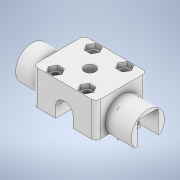
# Autodesk Inventor part: Part8
Saved by Autodesk Inventor 2022 (Build 260153000, 153)
## iProperties
Created: 2022-12-25
Part Number: Part8
Material: ABS Plastic
Document SubType Name: Modeling
Designer: Kamil
Density: 1.06 g/cm^3
Appearance: Smooth - White
Author: Kamil
Autodesk Inventor part; units mm, degrees
ref_plane "YZ Plane" through (0, 0, 0) normal (1, 0, 0) x (0, 1, 0)
ref_plane "XZ Plane" through (0, 0, 0) normal (0, 1, 0) x (-1, 0, 0)
ref_plane "XY Plane" through (0, 0, 0) normal (0, 0, 1) x (1, 0, 0)
ref_plane "Work Plane1" through (88.6183, 20.8479, 68.1697) normal (-1, 0, 0) x (0, 1, 0)
sketch "Sketch1" plane through (88.6183, 20.8479, 68.1697) normal (-1, 0, 0) x (0, 1, 0)
  arc A0 (4.3225, -4.9221) -> (4.3225, 4.9221) centre (-2.06, 0) ccw
  arc A1 (4.3225, -4.9221) -> (4.3225, 4.9221) centre (-2.06, 0) ccw
  arc A2 (4.3225, -4.9221) -> (4.3225, 4.9221) centre (-2.06, 0) ccw
  line L0 (-4.065, 4.6) -> (4.065, 4.6)
  arc A3 (4.065, -4.6) -> (4.065, 4.6) centre (-2.06, 0) ccw
  line L1 (4.065, -4.6) -> (-4.065, -4.6)
  arc A4 (-4.065, 4.6) -> (-4.065, -4.6) centre (2.06, 0) ccw
  circle A5 centre (0, 0) radius 1
  arc A6 (4.3225, -4.9221) -> (4.3225, 4.9221) centre (-2.06, 0) ccw
  arc A7 (4.3225, -4.9221) -> (4.3225, 4.9221) centre (-2.06, 0) ccw
  line L2 (-4.1641, 5) -> (4.1641, 5)
  arc A8 (5.9696, 0.6989) -> (4.3225, 4.9221) centre (-2.06, 0) ccw
  arc A9 (4.3225, 4.9221) -> (4.1641, 5) centre (4.1641, 4.8) ccw
  spline S0 degree 3 poles (-4.1641, 5) (-4.1596, 4.9818) (-4.1529, 4.9545) (-4.1346, 4.8801) (-4.1163, 4.8058) (-4.0908, 4.7033) (-4.065, 4.6) knots 0 0 0 0 0.5 0.5 0.5 1 1 1 1
  arc A10 (-4.3225, 4.9221) -> (-5.9696, 0.6989) centre (2.06, 0) ccw
  arc A11 (-4.1641, 5) -> (-4.3225, 4.9221) centre (-4.1641, 4.8) ccw
  line L3 (4.1641, -5) -> (-4.1641, -5)
  arc A12 (4.1641, -5) -> (4.3225, -4.9221) centre (4.1641, -4.8) ccw
  arc A13 (4.3225, -4.9221) -> (5.9244, -1.1011) centre (-2.06, 0) ccw
  arc A14 (-5.9244, -1.1011) -> (-4.3225, -4.9221) centre (2.06, 0) ccw
  arc A15 (-4.3225, -4.9221) -> (-4.1641, -5) centre (-4.1641, -4.8) ccw
  arc A16 (-5.9696, 0.6989) -> (-5.9244, -1.1011) centre (2.06, 0) ccw
  circle A17 centre (0, 0) radius 9.5
  line L4 (9.5, 0) -> (8.5, 0)
  line L5 (-6, 4) -> (-6, -4)
  arc A18 (-6, -4) -> (-5, -5) centre (-5, -4) ccw
  line L6 (-5, -5) -> (5, -5)
  arc A19 (5, -5) -> (6, -4) centre (5, -4) ccw
  line L7 (6, -4) -> (6, 4)
  arc A20 (6, 4) -> (5, 5) centre (5, 4) ccw
  line L8 (5, 5) -> (-5, 5)
  arc A21 (-5, 5) -> (-6, 4) centre (-5, 4) ccw
  circle A22 centre (-3, -2.5) radius 0.5
  circle A23 centre (0, 0) radius 0.5329
  line L9 (6, 4) -> (6, -4)
  arc A24 (6, 4) -> (5, 5) centre (5, 4) ccw
  line L10 (-5, 5) -> (5, 5)
  arc A25 (-5, 5) -> (-6, 4) centre (-5, 4) ccw
  line L11 (-6, -4) -> (-6, 4)
  arc A26 (-6, -4) -> (-5, -5) centre (-5, -4) ccw
  line L12 (5, -5) -> (-5, -5)
  arc A27 (5, -5) -> (6, -4) centre (5, -4) ccw
  circle A28 centre (0, 0) radius 1.5
  circle A29 centre (3.5, -2.5) radius 1.5
  circle A30 centre (-3.5, 2.5) radius 1.5
  circle A31 centre (4.5, 0) radius 0.625
  circle A32 centre (-4.5, 0) radius 0.625
  circle A33 centre (0, 0) radius 8.5
  line L13 (6, 4) -> (7.5, 4)
  line L14 (6, -4) -> (7.5, -4)
  line L15 (0, -9.5) -> (0, -7.9)
  circle A34 centre (0, 0) radius 7.9
  line L16 (5, -5) -> (5, -6.1164)
  line L17 (-5, -5) -> (-5, -6.1164)
  line L18 (-5, 5) -> (-5, 6.1164)
  line L19 (5, 5) -> (5, 6.1164)
  point P0 (-20.8479, 68.1697)
  point P1 (6.8125, -4)
  point P2 (6.8125, 4)
  dimension "d0" = 1
  dimension "d1" = 1.6
  constraints: 16 end point, 10 point on circle, 2 centre point, 2 coincident, 2 horizontal, 2 point on line, 2 vertical, 1 parallel
  measures "d0" distance of L4.start L4.end
  measures "d1" distance of L15.start L15.end
extrude "Extrusion1" add sketch "Sketch1" along normal blind 5 contours L6 L16 A34 L17 L3 | L7 L13 A34 L14 | L8 L2 L18 A34 L19
sketch "Sketch2" plane through (88.6183, 20.8479, 68.1697) normal (1, 0, 0) x (0, 0, -1)
  arc A0 (-6.1164, 5) -> (-6.1164, -5) centre (0, 0) ccw projected
  line L0 (-5, -5) -> (-6.1164, -5) projected
  line L1 (-5, 5) -> (-5, -5) projected
  line L2 (-6.1164, 5) -> (-5, 5) projected
  line L3 (4, 6.8125) -> (4, 6) projected
  arc A1 (4, 6.8125) -> (-4, 6.8125) centre (0, 0) ccw projected
  line L4 (-4, 6) -> (-4, 6.8125) projected
  line L5 (4, 6) -> (-4, 6) projected
  arc A2 (6.1164, -5) -> (6.1164, 5) centre (0, 0) ccw projected
  line L6 (5, 5) -> (6.1164, 5) projected
  line L7 (5, -5) -> (5, 5) projected
  line L8 (6.1164, -5) -> (5, -5) projected
  circle A3 centre (0, 0) radius 7.9
  line L9 (5, -5) -> (5, 5) projected
  arc A4 (5, 5) -> (4, 6) centre (4, 5) ccw projected
  line L10 (4, 6) -> (-4, 6) projected
  arc A5 (-4, 6) -> (-5, 5) centre (-4, 5) ccw projected
  line L11 (-5, 5) -> (-5, -5) projected
  arc A6 (-5, -5) -> (-4, -6) centre (-4, -5) ccw projected
  line L12 (-4, -6) -> (4, -6) projected
  arc A7 (4, -6) -> (5, -5) centre (4, -5) ccw projected
  circle A8 centre (2.5, -3.5) radius 1.75 projected
  circle A9 centre (-2.5, 3.5) radius 1.75 projected
  circle A10 centre (0, -4.5) radius 0.625 projected
  circle A11 centre (0, 4.5) radius 0.625 projected
  circle A12 centre (0, 0) radius 2 projected
  point P0 (68.1697, -20.8479)
  point P1 (6.1164, 5)
  point P2 (-4, 6.8125)
  constraints: 1 centre point, 1 coincident
ref_plane "Work Plane2" through (97.6183, 14.8479, 63.1697) normal (1, 0, 0) x (0, 1, 0)
extrude "Extrusion2" add sketch "Sketch2" along normal up to surface (9 mm away) contours L2 L1 L0 A0 | A3 L4 A5 L2 | A1 L3 L5 L4 | L8 L7 L6 A2 | A3 L6 A4 L3
sketch "Sketch3" plane through (83.6183, 20.8479, 68.1697) normal (-1, 0, 0) x (0, 0, 1)
  line L0 (6.1164, 5) -> (5, 5) projected
  arc A0 (6.1164, 5) -> (4, 6.8125) centre (0, 0) ccw projected
  line L1 (4, 6) -> (4, 6.8125) projected
  arc A1 (5, 5) -> (4, 6) centre (4, 5) ccw projected
  line L2 (-4, 6.8125) -> (-4, 6) projected
  arc A2 (-4, 6.8125) -> (-6.1164, 5) centre (0, 0) ccw projected
  line L3 (-5, 5) -> (-6.1164, 5) projected
  arc A3 (-4, 6) -> (-5, 5) centre (-4, 5) ccw projected
  point P0 (-68.1697, -20.8479)
extrude "Extrusion3" add sketch "Sketch3" against normal blind 10
sketch "Sketch4" plane through (88.6183, 20.8479, 68.1697) normal (-1, 0, 0) x (0, 1, 0)
  arc A0 (5.9696, 0.6989) -> (4.3225, 4.9221) centre (-2.06, 0) ccw projected
  arc A1 (4.3225, -4.9221) -> (5.9244, -1.1011) centre (-2.06, 0) ccw projected
  line L0 (4.1641, -5) -> (-4.1641, -5) projected
  line L1 (4.5, -1.1011) -> (4.5, 0.6989) projected
  line L2 (4.5, 0.6989) -> (5.9696, 0.6989) projected
  arc A2 (5.9696, 0.6989) -> (4.3225, 4.9221) centre (-2.06, 0) ccw projected
  arc A3 (4.3225, 4.9221) -> (4.1641, 5) centre (4.1641, 4.8) ccw projected
  line L3 (1, 5) -> (4.1641, 5) projected
  line L4 (1, 5) -> (1, -5) projected
  line L5 (1, -5) -> (4.1641, -5) projected
  arc A4 (4.1641, -5) -> (4.3225, -4.9221) centre (4.1641, -4.8) ccw projected
  arc A5 (4.3225, -4.9221) -> (5.9244, -1.1011) centre (-2.06, 0) ccw projected
  line L6 (5.9244, -1.1011) -> (4.5, -1.1011) projected
  arc A6 (-5, -6.1164) -> (-5, 6.1164) centre (0, 0) ccw projected
  line L7 (-5, 6.1164) -> (-5, 5) projected
  line L8 (-5, 5) -> (5, 5) projected
  arc A7 (6, 4) -> (5, 5) centre (5, 4) ccw projected
  line L9 (6, 4) -> (6, -4) projected
  arc A8 (5, -5) -> (6, -4) centre (5, -4) ccw projected
  line L10 (5, -5) -> (-5, -5) projected
  line L11 (-5, -5) -> (-5, -6.1164) projected
  arc A9 (5.9244, -1.1011) -> (5.9696, 0.6989) centre (-2.06, 0) ccw projected
  arc A10 (-4.3225, 4.9221) -> (-5.9696, 0.6989) centre (2.06, 0) ccw projected
  arc A11 (-5.9244, -1.1011) -> (-4.3225, -4.9221) centre (2.06, 0) ccw projected
  arc A12 (-5.9696, 0.6989) -> (-5.9244, -1.1011) centre (2.06, 0) ccw projected
  line L12 (-4.5, 0.6989) -> (-4.5, -1.1011) projected
  line L13 (-4.5, -1.1011) -> (-5.9244, -1.1011) projected
  arc A13 (-5.9244, -1.1011) -> (-4.3225, -4.9221) centre (2.06, 0) ccw projected
  arc A14 (-4.3225, -4.9221) -> (-4.1641, -5) centre (-4.1641, -4.8) ccw projected
  line L14 (-4.1641, -5) -> (-1, -5) projected
  line L15 (-1, 5) -> (-1, -5) projected
  line L16 (-4.1641, 5) -> (-1, 5) projected
  arc A15 (-4.1641, 5) -> (-4.3225, 4.9221) centre (-4.1641, 4.8) ccw projected
  arc A16 (-4.3225, 4.9221) -> (-5.9696, 0.6989) centre (2.06, 0) ccw projected
  line L17 (-5.9696, 0.6989) -> (-4.5, 0.6989) projected
  line L18 (-5, 5) -> (-5, -6.1164)
  point P0 (-20.8479, 68.1697)
  point P1 (-5, 3.8885)
  point P2 (-5, -3.8885)
  point P3 (-5, -5)
  point P4 (-4.1641, -5)
  point P5 (6, 0)
  point P6 (4.1641, 5)
  constraints: 2 end point
extrude "Extrusion4" add sketch "Sketch4" along normal up to surface (5 mm away) contours A0 A3 L8 A7 L9 A9 | L9 A8 L10 A4 A1 A9 | A15 A10 L18 L8 | L10 L18 A11 A14
ref_plane "Work Plane3" through (70.1183, 20.8479, 68.3708) normal (-1, 0, 0) x (0, 1, 0)
sketch "Sketch5" plane through (97.6183, 26.8479, 64.1697) normal (0, -1, 0) x (1, 0, 0)
  line L0 (-5.5, 8) -> (-5.5, 0) projected
  line L1 (-5.5, 8) -> (-4.5, 8) projected
  line L2 (-4.5, 8) -> (-4.5, 0) projected
  line L3 (-4.5, 0) -> (-5.5, 0) projected
  line L4 (-8, 0) -> (-8, 8) projected
  line L5 (-8, 8) -> (-9, 8) projected
  line L6 (-9, 0) -> (-9, 8) projected
  line L7 (-9, 0) -> (-8, 0) projected
  line L8 (-1, 8) -> (-1, 0) projected
  line L9 (-1, 0) -> (0, 0) projected
  line L10 (0, 8) -> (0, 0) projected
  line L11 (0, 8) -> (-1, 8) projected
  line L12 (0, 0) -> (-9, 0) projected
  line L13 (-5.6036, 0) -> (-7.8841, 0)
  line L14 (-7.8841, 0) -> (-7.8841, 1)
  line L15 (-7.8841, 1) -> (-5.6036, 1)
  line L16 (-5.6036, 1) -> (-5.6036, 0)
  line L17 (0, 8) -> (-9, 8) projected
  line L18 (-5.6036, 8) -> (-7.8841, 8)
  line L19 (-7.8841, 8) -> (-7.8841, 7)
  line L20 (-7.8841, 7) -> (-5.6036, 7)
  line L21 (-5.6036, 7) -> (-5.6036, 8)
  line L22 (-1.16, 0) -> (-4.2946, 0)
  line L23 (-4.2946, 0) -> (-4.2946, 1)
  line L24 (-4.2946, 1) -> (-1.16, 1)
  line L25 (-1.16, 1) -> (-1.16, 0)
  line L26 (-1.16, 8) -> (-4.2946, 8)
  line L27 (-4.2946, 8) -> (-4.2946, 7)
  line L28 (-4.2946, 7) -> (-1.16, 7)
  line L29 (-1.16, 7) -> (-1.16, 8)
  line L30 (0, -2.1164) -> (-14, -2.1164) projected
  line L31 (-1.16, 1) -> (-4.2946, 1)
  line L32 (-4.2946, 1) -> (-4.2946, -2.1164)
  line L33 (-4.2946, -2.1164) -> (-1.16, -2.1164)
  line L34 (-1.16, -2.1164) -> (-1.16, 1)
  line L35 (-5.6036, 1) -> (-7.8841, 1)
  line L36 (-7.8841, 1) -> (-7.8841, -2.1164)
  line L37 (-7.8841, -2.1164) -> (-5.6036, -2.1164)
  line L38 (-5.6036, -2.1164) -> (-5.6036, 1)
  line L39 (-14, 10.1164) -> (0, 10.1164) projected
  line L40 (-5.6036, 7) -> (-7.8841, 7)
  line L41 (-7.8841, 7) -> (-7.8841, 10.1164)
  line L42 (-7.8841, 10.1164) -> (-5.6036, 10.1164)
  line L43 (-5.6036, 10.1164) -> (-5.6036, 7)
  line L44 (-1.16, 7) -> (-4.2946, 7)
  line L45 (-4.2946, 7) -> (-4.2946, 10.1164)
  line L46 (-4.2946, 10.1164) -> (-1.16, 10.1164)
  line L47 (-1.16, 10.1164) -> (-1.16, 7)
  point P0 (-97.6183, -64.1697)
  point P1 (-1.16, 8)
  point P2 (-1.16, 10.1164)
  point P3 (-4.2946, 8)
  point P4 (-5.6036, 0)
  point P5 (-7.8841, 0)
  point P6 (-1.16, -2.1164)
  point P7 (-1.16, 0)
  point P8 (-4.2946, 0)
  dimension "d10" = 1
  dimension "d11" = 1
  constraints: 64 end point, 16 parallel, 10 point on line, 8 horizontal, 8 perpendicular
  measures "d10" distance between parallel lines of L12 L15
  measures "d11" distance of L19.end L18.end
extrude "Extrusion5" add sketch "Sketch5" along normal blind 0.5 contours L21 L20 L19 L17 | L17 L41 L39 L43 | L38 L30 L36 L12 | L12 L14 L15 L16 | L45 L39 L47 L17 | L17 L29 L28 L27 | L23 L24 L25 L12 | L12 L34 L30 L32
sketch "Sketch6" plane through (97.6183, 15.8479, 63.1697) normal (1, 0, 0) x (0, 0, -1)
  arc A0 (-9, 11) -> (-10, 10) centre (-9, 10) ccw projected
  line L0 (-1, 11) -> (-9, 11) projected
  arc A1 (0, 10) -> (-1, 11) centre (-1, 10) ccw projected
  line L1 (0, 0) -> (0, 10) projected
  line L2 (1.1164, 0) -> (0, 0) projected
  arc A2 (1.1164, 0) -> (-11.1164, 0) centre (-5, 5) ccw projected
  line L3 (-10, 0) -> (-11.1164, 0) projected
  line L4 (-10, 10) -> (-10, 0) projected
  arc A3 (-10.1391, 11) -> (-10.671, 10.5) centre (-5, 5) ccw projected
  line L5 (-10.1391, 11) -> (-11.1164, 11) projected
  line L6 (-11.1164, 11) -> (-11.1164, 10.5) projected
  line L7 (-10.671, 10.5) -> (-11.1164, 10.5) projected
  arc A4 (0.671, 10.5) -> (0.1391, 11) centre (-5, 5) ccw projected
  line L8 (1.1164, 10.5) -> (0.671, 10.5) projected
  line L9 (1.1164, 11) -> (1.1164, 10.5) projected
  line L10 (1.1164, 11) -> (0.1391, 11) projected
  point P0 (63.1697, -15.8479)
  point P1 (0.1391, 11)
  point P2 (0.671, 10.5)
  point P3 (-10.671, 10.5)
  point P4 (-10.1391, 11)
extrude "Extrusion6" cut sketch "Sketch6" against normal through all contours L7 L6 L5 A2 | A2 L10 L9 L8
sketch "Sketch7" plane through (83.6183, 20.8479, 68.1697) normal (-1, 0, 0) x (0, 0, 1)
  arc A0 (6.1164, -5) -> (-6.1164, -5) centre (0, 0) ccw projected
  line L0 (-6.1164, -5) -> (-3.8885, -5) projected
  arc A1 (-4.9221, -4.3225) -> (-3.8885, -5) centre (0, 2.06) ccw projected
  arc A2 (-5, -4.1641) -> (-4.9221, -4.3225) centre (-4.8, -4.1641) ccw projected
  line L1 (-5, -4.1641) -> (-5, 4.1641) projected
  arc A3 (-4.9221, 4.3225) -> (-5, 4.1641) centre (-4.8, 4.1641) ccw projected
  arc A4 (4.9221, 4.3225) -> (-4.9221, 4.3225) centre (0, -2.06) ccw projected
  arc A5 (5, 4.1641) -> (4.9221, 4.3225) centre (4.8, 4.1641) ccw projected
  line L2 (5, 4.1641) -> (5, -4.1641) projected
  arc A6 (4.9221, -4.3225) -> (5, -4.1641) centre (4.8, -4.1641) ccw projected
  arc A7 (3.8885, -5) -> (4.9221, -4.3225) centre (0, 2.06) ccw projected
  line L3 (6.1164, -5) -> (3.8885, -5) projected
  point P0 (-68.1697, -20.8479)
extrude "Extrusion7" cut sketch "Sketch7" against normal blind 1.5
sketch "Sketch8" plane through (85.1183, 20.8479, 68.1697) normal (-1, 0, 0) x (0, 0, 1)
  arc A0 (6.1164, -5) -> (-6.1164, -5) centre (0, 0) ccw projected
  line L0 (-3.8885, -5) -> (-6.1164, -5) projected
  arc A1 (-4.9221, -4.3225) -> (-3.8885, -5) centre (0, 2.06) ccw projected
  arc A2 (-5, -4.1641) -> (-4.9221, -4.3225) centre (-4.8, -4.1641) ccw projected
  line L1 (-5, 4.1641) -> (-5, -4.1641) projected
  arc A3 (-4.9221, 4.3225) -> (-5, 4.1641) centre (-4.8, 4.1641) ccw projected
  arc A4 (4.9221, 4.3225) -> (-4.9221, 4.3225) centre (0, -2.06) ccw projected
  arc A5 (5, 4.1641) -> (4.9221, 4.3225) centre (4.8, 4.1641) ccw projected
  line L2 (5, -4.1641) -> (5, 4.1641) projected
  arc A6 (4.9221, -4.3225) -> (5, -4.1641) centre (4.8, -4.1641) ccw projected
  arc A7 (3.8885, -5) -> (4.9221, -4.3225) centre (0, 2.06) ccw projected
  line L3 (6.1164, -5) -> (3.8885, -5) projected
  circle A8 centre (0, 0) radius 12.5 projected
  circle A9 centre (0, 0) radius 9.5 projected
  circle A10 centre (0, 0) radius 16.1 projected
  line L4 (-5, 4.1641) -> (-5, -4.1641) projected
  line L5 (-5, 0) -> (-8, 0)
  line L6 (-8, 0) -> (-8, 11.4896)
  line L7 (5, 0) -> (8, 0)
  arc A11 (4.9221, 4.3225) -> (0, 6) centre (0, -2.06) ccw projected
  line L8 (0, 6) -> (0, 9)
  line L9 (0, 9) -> (-8, 9)
  line L10 (8, 0) -> (8, 9.5)
  line L11 (0, 9) -> (8, 9)
  line L12 (-6.1164, -5) -> (6.1164, -5)
  line L13 (-6.1164, -5) -> (-10.7059, -5)
  line L14 (-10.7059, -5) -> (9.6672, -5)
  line L15 (-8, -1.0781) -> (-8, -5.1235)
  line L16 (8, 0) -> (8.0777, -5)
  line L17 (-8, 0) -> (-8, -1.0781)
  point P0 (-68.1697, -20.8479)
  point P1 (-8, -5)
  dimension "d18" = 3
  dimension "d19" = 3
  dimension "d20" = 3
  constraints: 26 end point, 6 point on line, 4 perpendicular, 3 horizontal, 2 midpoint, 2 point on circle, 2 vertical
  measures "d18" distance of L5.start L5.end
  measures "d19" distance of L7.start L7.end
  measures "d20" distance of L8.start L8.end
extrude "Extrusion8" add sketch "Sketch8" along normal up to surface (15 mm away) contours L3 A7 A6 L2 L7 A0 | A0 L7 L16 L14 | L7 L2 A5 A4 L8 A0 | A0 L8 L11 A9 L10 L7 | L8 A4 A3 L1 L5 A0 | A0 L5 L6 A9 L9 L8 | L0 A0 L5 L1 A2 A1 | A0 L13 L15 L17 L5 | A9 L11 L10 | A9 L6 L9
sketch "Sketch9" plane through (85.1183, 15.8479, 60.1697) normal (0, 0, -1) x (-1, 0, 0)
  line L0 (15, 0) -> (15, 14) projected
  line L1 (0, 14) -> (15, 14) projected
  line L2 (0, 14) -> (0, 0) projected
  line L3 (0, 0) -> (15, 0) projected
  point P0 (85.1183, -15.8479)
extrude "Extrusion9" add sketch "Sketch9" along normal blind 5
sketch "Sketch10" plane through (85.1183, 20.8479, 76.1697) normal (0, 0, 1) x (1, 0, 0)
  line L0 (-15, 9) -> (-15, 0) projected
  line L1 (0, 0) -> (-15, 0) projected
  line L2 (0, 0) -> (0, 9) projected
  line L3 (0, 9) -> (-15, 9) projected
  line L4 (-15, 0) -> (-15, -5) projected
  line L5 (0, -5) -> (-15, -5) projected
  line L6 (0, -5) -> (0, 0) projected
  line L7 (0, 0) -> (-15, 0) projected
  point P0 (-85.1183, -20.8479)
  point P1 (-15, 0)
extrude "Extrusion10" add sketch "Sketch10" along normal blind 5
sketch "Sketch11" plane through (70.1183, 29.8479, 55.1697) normal (0, 1, 0) x (1, 0, 0)
  line L0 (0, -8) -> (18.5, -8) projected
  line L1 (27.5, -8) -> (18.5, -8) projected
  line L2 (27.5, -8) -> (18.5, -8) projected
  line L3 (0, -8) -> (18.5, -8) projected
  line L4 (0, -18) -> (18.5, -18) projected
  line L5 (27.5, -18) -> (18.5, -18) projected
  line L6 (27.5, -18) -> (18.5, -18) projected
  line L7 (0, -18) -> (18.5, -18) projected
  line L8 (0, 0) -> (0, -26) projected
  line L9 (15, -26) -> (0, -26) projected
  line L10 (15, 0) -> (15, -26) projected
  line L11 (0, 0) -> (15, 0) projected
  line L12 (15, 0) -> (0, 0) projected
  line L13 (7.5, 0) -> (7.5, -8)
  line L14 (18.5, -17.9221) -> (0, -17.9221) projected
  circle A0 centre (7.5, -4) radius 1.65
  line L15 (15, 0) -> (15, -26) projected
  line L16 (0, -9.1115) -> (0, 0) projected
  line L17 (15, 0) -> (0, 0)
  line L18 (0, 0) -> (0, -0.3)
  line L19 (0, -0.3) -> (15, -0.3)
  line L20 (15, -0.3) -> (15, 0)
  line L21 (7.5, -4) -> (7.5, -0.8)
  line L22 (7.5, -0.8) -> (7.5, -7.2)
  line L23 (5.6525, -7.2) -> (3.805, -4)
  line L24 (3.805, -4) -> (5.6525, -0.8)
  line L25 (5.6525, -0.8) -> (9.3475, -0.8)
  line L26 (9.3475, -0.8) -> (11.195, -4)
  line L27 (11.195, -4) -> (9.3475, -7.2)
  line L28 (9.3475, -7.2) -> (5.6525, -7.2)
  line L29 (15, 0) -> (0, 0)
  line L30 (0, 0) -> (0, -0.8)
  line L31 (0, -0.8) -> (15, -0.8)
  line L32 (15, -0.8) -> (15, 0)
  line L33 (0, -26) -> (15, -26) projected
  line L34 (7.5, -26) -> (7.5, -18)
  line L35 (0, -18) -> (18.5, -18) projected
  circle A1 centre (7.5, -22) radius 1.65
  line L36 (3.805, -22) -> (5.6525, -18.8)
  line L37 (5.6525, -18.8) -> (9.3475, -18.8)
  line L38 (9.3475, -18.8) -> (11.195, -22)
  line L39 (11.195, -22) -> (9.3475, -25.2)
  line L40 (9.3475, -25.2) -> (5.6525, -25.2)
  line L41 (5.6525, -25.2) -> (3.805, -22)
  line L42 (0, -16.8885) -> (0, -26) projected
  line L43 (0, -26) -> (15, -26)
  line L44 (15, -26) -> (15, -25.2)
  line L45 (15, -25.2) -> (0, -25.2)
  line L46 (0, -25.2) -> (0, -26)
  point P0 (-70.1183, 55.1697)
  point P1 (9.3475, -0.8)
  point P2 (15, -0.8)
  point P3 (0, -0.8)
  point P4 (5.6525, -0.8)
  point P5 (15, -25.2)
  point P6 (9.3475, -25.2)
  point P7 (5.6525, -25.2)
  point P8 (0, -25.2)
  point P9 (5.6525, -25.2)
  point P10 (9.3475, -25.2)
  point P11 (9.3475, -0.8)
  point P12 (5.6525, -0.8)
  dimension "d27" = 3.3
  dimension "d28" = 0.3
  dimension "d29" = 3.2
  dimension "d30" = 6.4
  constraints: 56 end point, 7 point on line, 6 parallel, 5 midpoint, 5 perpendicular, 3 horizontal, 2 centre point, 2 coincident, 26 other
  measures "d27" diameter of A0
  measures "d28" distance of L18.end L17.end
  measures "d29" distance of L21.start L21.end
  measures "d30" distance of L21.end L22.end
extrude "Extrusion11" cut sketch "Sketch11" against normal through all contours L8 L19 L13 L25 L31 | L8 L11 L13 L19 | L31 L25 L13 L19 L10 | A0 L13 | L13 A0 | L13 L11 L10 L19 | L10 L9 L34 L40 L45 | L45 L40 L34 L9 L8 | A1 L34 | L34 A1
extrude "Extrusion12" add sketch "Sketch11" along normal blind 2 contours L8 L31 L24 L23 L28 L13 L0 | L0 L10 L14 L8 | L13 L28 L27 L26 L31 L10 L0 | L10 L4 L8 L14 | L10 L45 L39 L38 L37 L34 L4 | L4 L34 L37 L36 L41 L45 L8
sketch "Sketch12" plane through (75.7708, 29.8479, 73.9697) normal (0, 1, 0) x (1, 0, 0)
  circle A0 centre (1.8475, -3.2) radius 1.65 projected
  circle A1 centre (1.8475, 14.8) radius 1.65 projected
  circle A2 centre (1.8475, -3.2) radius 1.65 projected
  circle A3 centre (1.8475, -3.2) radius 1.75
  circle A4 centre (1.8475, 14.8) radius 1.65 projected
  circle A5 centre (1.8475, 14.8) radius 1.75
  point P0 (-75.7708, 73.9697)
  dimension "d35" = 3.5
  dimension "d36" = 3.5
  constraints: 2 centre point, 2 coincident
  measures "d35" diameter of A3
  measures "d36" diameter of A5
extrude "Extrusion13" cut sketch "Sketch12" against normal through all contours A0 | A1 | A3 | A5
sketch "Sketch13" plane through (70.1183, 31.8479, 55.1697) normal (0, 1, 0) x (1, 0, 0)
  line L0 (0, -25.2) -> (5.6525, -25.2) projected
  line L1 (5.6525, -25.2) -> (3.805, -22) projected
  line L2 (3.805, -22) -> (5.6525, -18.8) projected
  line L3 (5.6525, -18.8) -> (9.3475, -18.8) projected
  line L4 (9.3475, -18.8) -> (11.195, -22) projected
  line L5 (11.195, -22) -> (9.3475, -25.2) projected
  line L6 (9.3475, -25.2) -> (15, -25.2) projected
  line L7 (15, -25.2) -> (15, -0.8) projected
  line L8 (15, -0.8) -> (9.3475, -0.8) projected
  line L9 (9.3475, -0.8) -> (11.195, -4) projected
  line L10 (11.195, -4) -> (9.3475, -7.2) projected
  line L11 (9.3475, -7.2) -> (5.6525, -7.2) projected
  line L12 (5.6525, -7.2) -> (3.805, -4) projected
  line L13 (3.805, -4) -> (5.6525, -0.8) projected
  line L14 (5.6525, -0.8) -> (0, -0.8) projected
  line L15 (0, -0.8) -> (0, -25.2) projected
  line L16 (0, -8) -> (18.5, -8) projected
  line L17 (27.5, -8) -> (18.5, -8) projected
  line L18 (27.5, -8) -> (18.5, -8) projected
  line L19 (0, -8) -> (18.5, -8) projected
  line L20 (0, -0.8) -> (0, -25.2) projected
  circle A0 centre (0, -13) radius 2.6186
  point P0 (-70.1183, 55.1697)
  point P1 (0, -10.3814)
  point P2 (0, -15.6186)
  constraints: 1 centre point, 1 midpoint
extrude "Extrusion14" cut sketch "Sketch13" against normal blind 10 contours L15 A0 picked at (0.5442, -12.3176)
mirror "Mirror1" about plane through (70.1183, 20.8479, 68.3708) normal (-1, 0, 0)
fillet "Fillet1" radius 2 10 edges at (85.1183, 30.8479, 55.9697) (85.1183, 22.8479, 55.9697) (55.1183, 30.8479, 55.9697) (55.1183, 22.8479, 55.9697) (85.1183, 30.8479, 80.3697) (85.1183, 25.3479, 80.3697) (85.1183, 18.3479, 80.3697) (55.1183, 30.8479, 80.3697) (55.1183, 25.3479, 80.3697) (55.1183, 18.3479, 80.3697)
sketch "Sketch14" plane through (88.6183, 15.8479, 73.1697) normal (0, -1, 0) x (1, 0, 0)
  arc A0 (-31.5, 7.2) -> (-33.5, 5.2) centre (-31.5, 5.2) ccw projected
  line L0 (-33.5, 1.1164) -> (-33.5, 5.2) projected
  line L1 (-33.5, 1.1164) -> (-46, 1.1164) projected
  line L2 (-46, 0) -> (-46, 1.1164) projected
  line L3 (-46, 0) -> (-37, 0) projected
  line L4 (-37, -1.1115) -> (-37, 0) projected
  line L5 (0, -1.1115) -> (-37, -1.1115) projected
  line L6 (0, -1.1115) -> (0, 0) projected
  line L7 (9, 0) -> (0, 0) projected
  line L8 (9, 0) -> (9, 1.1164) projected
  line L9 (-3.5, 1.1164) -> (9, 1.1164) projected
  line L10 (-3.5, 1.1164) -> (-3.5, 5.2) projected
  arc A1 (-3.5, 5.2) -> (-5.5, 7.2) centre (-5.5, 5.2) ccw projected
  line L11 (-5.5, 7.2) -> (-31.5, 7.2) projected
  circle A2 centre (-26, 4) radius 1.75 projected
  circle A3 centre (-11, 4) radius 1.75 projected
  arc A4 (-33.5, -15.2) -> (-31.5, -17.2) centre (-31.5, -15.2) ccw projected
  line L12 (-5.5, -17.2) -> (-31.5, -17.2) projected
  arc A5 (-5.5, -17.2) -> (-3.5, -15.2) centre (-5.5, -15.2) ccw projected
  line L13 (-3.5, -11.1164) -> (-3.5, -15.2) projected
  line L14 (9, -11.1164) -> (-3.5, -11.1164) projected
  line L15 (9, -11.1164) -> (9, -10) projected
  line L16 (9, -10) -> (0, -10) projected
  line L17 (0, -10) -> (0, -8.8885) projected
  line L18 (0, -8.8885) -> (-37, -8.8885) projected
  line L19 (-37, -10) -> (-37, -8.8885) projected
  line L20 (-46, -10) -> (-37, -10) projected
  line L21 (-46, -11.1164) -> (-46, -10) projected
  line L22 (-46, -11.1164) -> (-33.5, -11.1164) projected
  line L23 (-33.5, -11.1164) -> (-33.5, -15.2) projected
  circle A6 centre (-26, -14) radius 1.75 projected
  circle A7 centre (-11, -14) radius 1.75 projected
  line L24 (-3.5, 1.1164) -> (9, 1.1164) projected
  line L25 (-3.5, 1.1164) -> (-3.5, -1.1115)
  line L26 (9, -11.1164) -> (-3.5, -11.1164) projected
  line L27 (-3.5, -8.8885) -> (-3.5, -11.1164)
  line L28 (-33.5, -11.1164) -> (-33.5, 1.1164)
  point P0 (-88.6183, -73.1697)
  point P1 (-33.5, -8.8885)
  point P2 (-33.5, -1.1115)
  constraints: 6 end point, 3 point on line, 2 perpendicular, 1 vertical
extrude "Extrusion15" add sketch "Sketch14" along normal blind 0.9185 contours L11 A1 L10 L25 L5 L28 L0 A0 | L23 L28 L18 L27 L13 A5 L12 A4
sketch "Sketch15" plane through (75.7708, 29.8479, 80.3697) normal (0, 0, 1) x (1, 0, 0)
  line L0 (-18.6525, -14.9185) -> (-18.6525, 2) projected
  line L1 (7.3475, -14.9185) -> (-18.6525, -14.9185) projected
  line L2 (7.3475, 2) -> (7.3475, -14.9185) projected
  line L3 (3.695, 2) -> (7.3475, 2) projected
  line L4 (3.695, 0) -> (3.695, 2) projected
  line L5 (0, 0) -> (3.695, 0) projected
  line L6 (0, 0) -> (0, 2) projected
  line L7 (0, 2) -> (-11.305, 2) projected
  line L8 (-11.305, 0) -> (-11.305, 2) projected
  line L9 (-11.305, 0) -> (-15, 0) projected
  line L10 (-15, 0) -> (-15, 2) projected
  line L11 (-15, 2) -> (-18.6525, 2) projected
  line L12 (-3.0339, 2) -> (-8.2711, 2) projected
  line L13 (-5.6525, 2) -> (-5.6525, -14.9185)
  line L14 (-8.0525, -12.6889) -> (-9.1525, -12.6889) projected
  line L15 (-8.0525, -5.3111) -> (-9.1525, -5.3111) projected
  line L16 (-8.0525, -12.6889) -> (-9.1525, -12.6889) projected
  line L17 (-5.6525, -5.7296) -> (-5.6525, -13.1074)
  circle A0 centre (-5.6525, -9.4185) radius 4.1641
  line L18 (-9.8166, -9.4185) -> (-9.8166, -14.9185)
  line L19 (7.3475, -14.9185) -> (-18.6525, -14.9185) projected
  line L20 (-1.4884, -9.4185) -> (-1.4884, -14.9185)
  point P0 (-75.7708, -29.8479)
  constraints: 8 end point, 4 point on line, 3 midpoint, 2 point on circle, 1 centre point, 1 perpendicular, 1 vertical
extrude "Extrusion16" cut sketch "Sketch15" against normal blind 9 contours L18 A0 L13 L1 | L13 A0 L20 L1 | A0 L13 | L13 A0
sketch "Sketch16" plane through (88.6183, 14.9294, 73.1697) normal (0, -1, 0) x (1, 0, 0)
  line L0 (-22.6641, -1.1115) -> (-22.6641, 7.2) projected
  line L1 (-22.6641, 7.2) -> (-31.5, 7.2) projected
  arc A0 (-31.5, 7.2) -> (-33.5, 5.2) centre (-31.5, 5.2) ccw projected
  line L2 (-33.5, 5.2) -> (-33.5, -1.1115) projected
  line L3 (-33.5, -1.1115) -> (-22.6641, -1.1115) projected
  circle A1 centre (-26, 4) radius 1.75 projected
  circle A2 centre (-11, 4) radius 1.75 projected
  line L4 (-14.3359, 7.2) -> (-14.3359, -1.1115) projected
  line L5 (-14.3359, -1.1115) -> (-3.5, -1.1115) projected
  line L6 (-3.5, -1.1115) -> (-3.5, 5.2) projected
  arc A3 (-3.5, 5.2) -> (-5.5, 7.2) centre (-5.5, 5.2) ccw projected
  line L7 (-5.5, 7.2) -> (-14.3359, 7.2) projected
  line L8 (-3.5, -15.2) -> (-3.5, -8.8885) projected
  line L9 (-3.5, -8.8885) -> (-33.5, -8.8885) projected
  line L10 (-33.5, -8.8885) -> (-33.5, -15.2) projected
  arc A4 (-33.5, -15.2) -> (-31.5, -17.2) centre (-31.5, -15.2) ccw projected
  line L11 (-31.5, -17.2) -> (-5.5, -17.2) projected
  arc A5 (-5.5, -17.2) -> (-3.5, -15.2) centre (-5.5, -15.2) ccw projected
  circle A6 centre (-11, -14) radius 1.75 projected
  circle A7 centre (-26, -14) radius 1.75 projected
  point P0 (-88.6183, -73.1697)
extrude "Extrusion17" cut sketch "Sketch16" against normal blind 0.5
sketch "Sketch17" plane through (70.1183, 31.8479, 55.1697) normal (0, 1, 0) x (1, 0, 0)
  circle A0 centre (0, -13) radius 2.6186 projected
  arc A1 (-15, -23.2) -> (-13, -25.2) centre (-13, -23.2) ccw projected
  line L0 (-9.3475, -25.2) -> (-13, -25.2) projected
  line L1 (-11.195, -22) -> (-9.3475, -25.2) projected
  line L2 (-9.3475, -18.8) -> (-11.195, -22) projected
  line L3 (-5.6525, -18.8) -> (-9.3475, -18.8) projected
  line L4 (-3.805, -22) -> (-5.6525, -18.8) projected
  line L5 (-5.6525, -25.2) -> (-3.805, -22) projected
  line L6 (5.6525, -25.2) -> (-5.6525, -25.2) projected
  line L7 (5.6525, -25.2) -> (3.805, -22) projected
  line L8 (3.805, -22) -> (5.6525, -18.8) projected
  line L9 (5.6525, -18.8) -> (9.3475, -18.8) projected
  line L10 (9.3475, -18.8) -> (11.195, -22) projected
  line L11 (11.195, -22) -> (9.3475, -25.2) projected
  line L12 (9.3475, -25.2) -> (13, -25.2) projected
  arc A2 (13, -25.2) -> (15, -23.2) centre (13, -23.2) ccw projected
  line L13 (15, -23.2) -> (15, -2.8) projected
  arc A3 (15, -2.8) -> (13, -0.8) centre (13, -2.8) ccw projected
  line L14 (13, -0.8) -> (9.3475, -0.8) projected
  line L15 (9.3475, -0.8) -> (11.195, -4) projected
  line L16 (11.195, -4) -> (9.3475, -7.2) projected
  line L17 (9.3475, -7.2) -> (5.6525, -7.2) projected
  line L18 (5.6525, -7.2) -> (3.805, -4) projected
  line L19 (3.805, -4) -> (5.6525, -0.8) projected
  line L20 (5.6525, -0.8) -> (-5.6525, -0.8) projected
  line L21 (-3.805, -4) -> (-5.6525, -0.8) projected
  line L22 (-5.6525, -7.2) -> (-3.805, -4) projected
  line L23 (-9.3475, -7.2) -> (-5.6525, -7.2) projected
  line L24 (-11.195, -4) -> (-9.3475, -7.2) projected
  line L25 (-9.3475, -0.8) -> (-11.195, -4) projected
  line L26 (-13, -0.8) -> (-9.3475, -0.8) projected
  arc A4 (-13, -0.8) -> (-15, -2.8) centre (-13, -2.8) ccw projected
  line L27 (-15, -23.2) -> (-15, -2.8) projected
  line L28 (0, -13) -> (15, -13)
  line L29 (0, -13) -> (0, -0.8)
  circle A5 centre (7.5, -4) radius 1.75 projected
  line L30 (7.5, -4) -> (7.5, -1.25)
  line L31 (9.0877, -1.25) -> (10.6754, -4)
  line L32 (10.6754, -4) -> (9.0877, -6.75)
  line L33 (9.0877, -6.75) -> (5.9123, -6.75)
  line L34 (5.9123, -6.75) -> (4.3246, -4)
  line L35 (4.3246, -4) -> (5.9123, -1.25)
  line L36 (5.9123, -1.25) -> (9.0877, -1.25)
  line L37 (9.3475, -0.8) -> (5.6525, -0.8) projected
  line L38 (-13, -0.8) -> (-9.3475, -0.8)
  line L39 (-9.3475, -0.8) -> (-11.195, -4)
  line L40 (-11.195, -4) -> (-9.3475, -7.2)
  line L41 (-9.3475, -7.2) -> (-5.6525, -7.2)
  line L42 (-5.6525, -7.2) -> (-3.805, -4)
  line L43 (-3.805, -4) -> (-5.6525, -0.8)
  line L44 (-5.6525, -0.8) -> (5.6525, -0.8)
  circle A6 centre (-7.5, -4) radius 1.75
  line L45 (-7.5, -4) -> (-7.5, -1.25)
  line L46 (-9.0877, -1.25) -> (-10.6754, -4)
  line L47 (-10.6754, -4) -> (-9.0877, -6.75)
  line L48 (-9.0877, -6.75) -> (-5.9123, -6.75)
  line L49 (-5.9123, -6.75) -> (-4.3246, -4)
  line L50 (-4.3246, -4) -> (-5.9123, -1.25)
  line L51 (-5.9123, -1.25) -> (-9.0877, -1.25)
  line L52 (-9.3475, -0.8) -> (-5.6525, -0.8)
  line L53 (13, -25.2) -> (9.3475, -25.2)
  line L54 (9.3475, -25.2) -> (11.195, -22)
  line L55 (11.195, -22) -> (9.3475, -18.8)
  line L56 (9.3475, -18.8) -> (5.6525, -18.8)
  line L57 (5.6525, -18.8) -> (3.805, -22)
  line L58 (3.805, -22) -> (5.6525, -25.2)
  line L59 (5.6525, -25.2) -> (-5.6525, -25.2)
  line L60 (-3.805, -22) -> (-5.6525, -25.2)
  line L61 (-5.6525, -18.8) -> (-3.805, -22)
  line L62 (-9.3475, -18.8) -> (-5.6525, -18.8)
  line L63 (-11.195, -22) -> (-9.3475, -18.8)
  line L64 (-9.3475, -25.2) -> (-11.195, -22)
  line L65 (-13, -25.2) -> (-9.3475, -25.2)
  line L66 (0, -13) -> (0, -25.2)
  circle A7 centre (7.5, -22) radius 1.75
  line L67 (7.5, -22) -> (7.5, -24.75)
  line L68 (9.0877, -24.75) -> (10.6754, -22)
  line L69 (10.6754, -22) -> (9.0877, -19.25)
  line L70 (9.0877, -19.25) -> (5.9123, -19.25)
  line L71 (5.9123, -19.25) -> (4.3246, -22)
  line L72 (4.3246, -22) -> (5.9123, -24.75)
  line L73 (5.9123, -24.75) -> (9.0877, -24.75)
  line L74 (9.3475, -25.2) -> (5.6525, -25.2)
  line L75 (-10.6754, -22) -> (-9.0877, -19.25)
  line L76 (-9.0877, -19.25) -> (-5.9123, -19.25)
  line L77 (-5.6525, -18.8) -> (-3.805, -22)
  line L78 (-9.3475, -18.8) -> (-5.6525, -18.8)
  line L79 (-11.195, -22) -> (-9.3475, -18.8)
  line L80 (-5.9123, -19.25) -> (-4.3246, -22)
  line L81 (-5.6525, -25.2) -> (5.6525, -25.2)
  circle A8 centre (-7.5, -22) radius 1.75
  line L82 (-13, -25.2) -> (-9.3475, -25.2)
  line L83 (-9.0877, -24.75) -> (-10.6754, -22)
  line L84 (-9.3475, -25.2) -> (-11.195, -22)
  line L85 (-4.3246, -22) -> (-5.9123, -24.75)
  line L86 (-7.5, -22) -> (-7.5, -24.75)
  line L87 (-3.805, -22) -> (-5.6525, -25.2)
  line L88 (-5.9123, -24.75) -> (-9.0877, -24.75)
  line L89 (-9.3475, -25.2) -> (-5.6525, -25.2)
  point P0 (-70.1183, 55.1697)
  dimension "d48" = 2.75
  constraints: 122 end point, 34 symmetric about line, 4 coincident, 3 centre point, 3 midpoint, 1 vertical, 16 other
  measures "d48" distance of L30.start L30.end
extrude "Extrusion18" add sketch "Sketch17" against normal up to surface (2 mm away) contours L37 L15 L16 L17 L18 L19 | L21 L22 L23 L24 L25 L52 | L7 L8 L9 L10 L11 L74 | L89 L1 L2 L3 L4 L5
body "Solid1"
